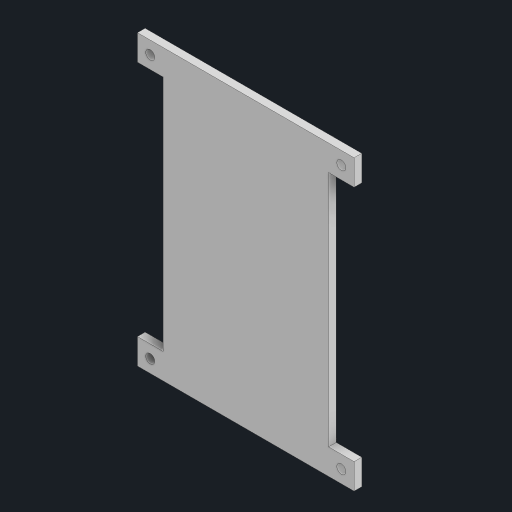
# Autodesk Inventor part: CAJA_P2
Saved by Autodesk Inventor 2024.3 (Build 283343000, 343)
## iProperties
Created: 2024-07-22
Part Number: CAJA_P2
Material: Generic
Document SubType Name: Modeling
Designer: Niler
Density: 1 g/cm^3
Appearance: Default
Author: Niler
Autodesk Inventor part; units mm, degrees
ref_plane "YZ Plane" through (0, 0, 0) normal (1, 0, 0) x (0, 1, 0)
ref_plane "XZ Plane" through (0, 0, 0) normal (0, 1, 0) x (-1, 0, 0)
ref_plane "XY Plane" through (0, 0, 0) normal (0, 0, 1) x (1, 0, 0)
sketch "Sketch1" plane through (0, 0, 0) normal (0, 0, 1) x (1, 0, 0)
  circle A0 centre (37.4, -51.5) radius 1.75 projected
  circle A1 centre (37.4, 51.5) radius 1.75 projected
  circle A2 centre (-37.4, -51.5) radius 1.75 projected
  circle A3 centre (-37.4, 51.5) radius 1.75 projected
  line L0 (-32.4, 46.5) -> (-32.4, -46.5) projected
  line L1 (-32.4, -46.5) -> (-42.4, -46.5) projected
  line L2 (-42.4, -46.5) -> (-42.4, -56.5) projected
  line L3 (-42.4, -56.5) -> (42.4, -56.5) projected
  line L4 (42.4, -56.5) -> (42.4, -46.5) projected
  line L5 (42.4, -46.5) -> (32.4, -46.5) projected
  line L6 (32.4, -46.5) -> (32.4, 46.5) projected
  line L7 (32.4, 46.5) -> (42.4, 46.5) projected
  line L8 (42.4, 46.5) -> (42.4, 56.5) projected
  line L9 (42.4, 56.5) -> (-42.4, 56.5) projected
  line L10 (-42.4, 56.5) -> (-42.4, 46.5) projected
  line L11 (-42.4, 46.5) -> (-32.4, 46.5) projected
  line L12 (30.4, -54.5) -> (-30.4, -54.5) projected
  line L13 (-30.4, -54.5) -> (-30.4, 54.5) projected
  line L14 (-30.4, 54.5) -> (30.4, 54.5) projected
  line L15 (30.4, 54.5) -> (30.4, -54.5) projected
  point P0 (0, 0)
extrude "Extrusion1" add sketch "Sketch1" along normal blind 3 contours L11 L10 L9 L8 L7 L6 L5 L4 L3 L2 L1 L0 | L12 L13 L14 L15
sketch "Sketch2" plane through (0, 0, 0) normal (0, 0, -1) x (-1, 0, 0)
  circle A0 centre (26.3, -50.4) radius 1.5 projected
  circle A1 centre (-26.3, -50.4) radius 1.5 projected
  circle A2 centre (-26.3, 50.4) radius 1.5 projected
  circle A3 centre (26.3, 50.4) radius 1.5 projected
  circle A4 centre (26.3, -50.4) radius 1.25
  circle A5 centre (-26.3, -50.4) radius 1.25
  circle A6 centre (-26.3, 50.4) radius 1.25
  circle A7 centre (26.3, 50.4) radius 1.25
  circle A8 centre (-26.3, -50.4) radius 2
  circle A9 centre (26.3, -50.4) radius 2
  circle A10 centre (26.3, 50.4) radius 2
  circle A11 centre (-26.3, 50.4) radius 2
  point P0 (0, 0)
  dimension "d2" = 2.5
  dimension "d3" = 4
  constraints: 8 centre point, 8 coincident, 6 equal radius
  measures "d2" diameter of A4
  measures "d3" diameter of A8
extrude "Extrusion2" add sketch "Sketch2" along normal blind 2.1 contours A0 | A1 | A2 | A3 | A8 | A9 | A10 | A11
fillet "Fillet1" radius 1.5 4 edges at (28.3, -50.4, 0) (-24.3, -50.4, 0) (-24.3, 50.4, 0) (28.3, 50.4, 0)
sketch "Sketch3" plane through (-26.3, -50.4, 0) normal (0, 0, -1) x (-1, 0, 0)
  circle A0 centre (0, 0) radius 2 projected
  circle A1 centre (0, 0) radius 1.25 projected
  circle A2 centre (-52.6, 0) radius 1.25 projected
  circle A3 centre (-52.6, 100.8) radius 1.25 projected
  circle A4 centre (0, 100.8) radius 1.25 projected
  point P0 (-26.3, 50.4)
extrude "Extrusion3" add sketch "Sketch3" along normal blind 5 contours A1 | A2 | A3 | A4
body "Solid1"
